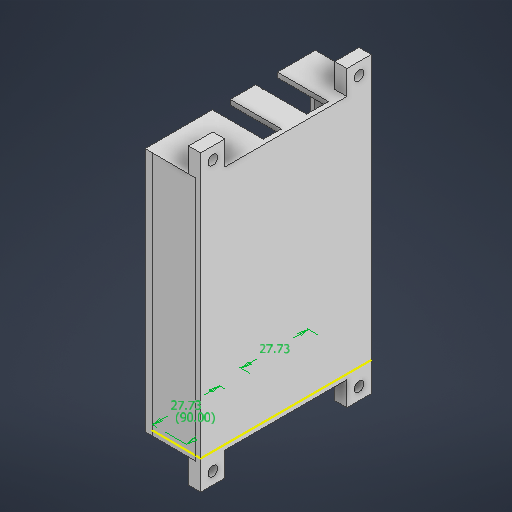
# Autodesk Inventor part: SAFRS-P-0019
Saved by Autodesk Inventor 2026.2 (Build 302298000, 298)
## iProperties
Created: 2025-11-19
Part Number: SAFRS-P-0019
Material: Generic
Document SubType Name: Modeling
Designer: ost97
Density: 1 g/cm^3
Appearance: Default
Author: ost97
Title: STM32 Board
Autodesk Inventor part; units mm, degrees
ref_plane "YZ Plane" through (0, 0, 0) normal (1, 0, 0) x (0, 1, 0)
ref_plane "XZ Plane" through (0, 0, 0) normal (0, 1, 0) x (-1, 0, 0)
ref_plane "XY Plane" through (0, 0, 0) normal (0, 0, 1) x (1, 0, 0)
sketch "Sketch1" plane through (0, 0, 0) normal (0, 1, 0) x (-1, 0, 0)
  line L0 (15, 35.0917) -> (15, 35.175)
  line L1 (-2, 35.175) -> (-2, -33.075)
  line L2 (-2, -33.075) -> (-2, -35.075)
  line L3 (15, 33.075) -> (15, 28.875)
  line L4 (15, 28.875) -> (0, 28.875)
  line L5 (15, 33.075) -> (18, 33.075)
  line L6 (18, 33.075) -> (18, 35.075)
  line L7 (18, 35.075) -> (0, 35.175)
  line L8 (15, -33.075) -> (15, -28.875)
  line L9 (15, -28.875) -> (0, -28.875)
  line L10 (15, -33.075) -> (18, -33.075)
  line L11 (18, -33.075) -> (18, -35.075)
  line L12 (18, -35.075) -> (0, -35.075)
  line L13 (0, 35.175) -> (-2, 35.175)
  line L14 (0, -35.075) -> (-2, -35.075)
  line L15 (0, 28.875) -> (0, -28.875)
  point P0 (0, 0)
  point P1 (15, 39.275)
  point P2 (-2, -37.275)
  point P3 (-2, -39.275)
  point P4 (18, -39.275)
  point P5 (18, -37.275)
  constraints: 32 end point, 7 perpendicular, 5 point on line, 2 horizontal, 2 vertical, 1 midpoint
extrude "Extrusion1" add sketch "Sketch1" against normal blind 97
sketch "Sketch2" plane through (0, 0, 0) normal (0, 1, 0) x (1, 0, 0)
  line L0 (2, 39.275) -> (-18, 39.275) projected
  line L1 (2, -35.175) -> (2, 35.075) projected
  line L2 (-18, 39.275) -> (-18, 37.275) projected
  line L3 (-18, 35.075) -> (-18, 25.675)
  line L4 (0, -28.875) -> (0, 28.875) projected
  line L5 (0, 25.675) -> (0, 17.695)
  line L6 (-18.0003, 10.5) -> (-18.0012, 7.2)
  line L7 (-18, -35.075) -> (-18.0067, -12.57)
  line L8 (-18, -33.075) -> (-18, -35.075) projected
  line L9 (-18, -35.075) -> (0, -35.175) projected
  line L10 (2, 35.075) -> (-18, 35.075) projected
  line L11 (-18, 35.075) -> (-18, 33.075) projected
  line L12 (-18, -35.075) -> (-18, -33.075) projected
  line L13 (-18, -35.075) -> (-18, -10.375)
  line L14 (-18, 33.075) -> (-18, 19.475)
  line L15 (-18, 19.475) -> (0, 19.475)
  line L16 (0, 19.475) -> (0, 11.495)
  line L17 (-18, 10.5) -> (-18, 1)
  line L18 (-18, -33.075) -> (-18.0079, -8.375)
  line L19 (-18.0079, -8.375) -> (0, -8.375)
  line L20 (0, 11.495) -> (0, 10.495)
  line L21 (0, 10.495) -> (-18, 10.5)
  line L22 (-18, 1) -> (-18, 0)
  line L23 (-18, 0) -> (0, 0)
  line L24 (0, -35.175) -> (-18, -35.075) projected
  line L25 (-18, -33.075) -> (-15, -33.075) projected
  line L26 (-18, -35.075) -> (0, -35.175) projected
  line L27 (0, -35.175) -> (2, -35.175) projected
  line L28 (2, -35.175) -> (2, 35.075) projected
  line L29 (2, 35.075) -> (-18, 35.075) projected
  line L30 (-18, 35.075) -> (-18, 33.075) projected
  line L31 (-18, 33.075) -> (-15, 33.075) projected
  line L32 (-15, 33.075) -> (-15, 28.875) projected
  line L33 (-15, 28.875) -> (0, 28.875) projected
  line L34 (0, 28.875) -> (0, -28.875) projected
  line L35 (0, -28.875) -> (-15, -28.875) projected
  line L36 (-15, -28.875) -> (-15, -33.075) projected
  line L37 (-15, -33.075) -> (-18, -33.075) projected
  line L38 (-18, -33.075) -> (-18, -35.075) projected
  line L39 (2, -35.175) -> (2, 35.075) projected
  line L40 (2, 35.075) -> (2, -35.175) projected
  line L41 (-15, -33.075) -> (-18, -33.075) projected
  line L42 (-15, -28.875) -> (-15, -33.075) projected
  line L43 (0, -28.875) -> (-15, -28.875) projected
  line L44 (0, 28.875) -> (0, -28.875) projected
  line L45 (0, 28.875) -> (0, -28.875) projected
  line L46 (0, -28.875) -> (0, 28.875) projected
  line L47 (2, 35.075) -> (-18, 35.075) projected
  line L48 (-18, 35.075) -> (2, 35.075) projected
  line L49 (-15, 28.875) -> (0, 28.875) projected
  line L50 (-15, 28.875) -> (0, 28.875) projected
  line L51 (0, 28.875) -> (-15, 28.875) projected
  line L52 (-15, 33.075) -> (-15, 28.875) projected
  line L53 (-15, 33.075) -> (-15, 28.875) projected
  line L54 (-15, 28.875) -> (-15, 33.075) projected
  line L55 (-18, 35.075) -> (-18, 33.075) projected
  line L56 (-18, 33.075) -> (-18, 35.075) projected
  line L57 (-18, 33.075) -> (-15, 33.075) projected
  line L58 (-15, 33.075) -> (-18, 33.075) projected
  line L59 (-18, 33.075) -> (-15, 33.075) projected
  line L60 (-15, 33.075) -> (-18, 33.075) projected
  line L61 (-18, 33.075) -> (-18, 35.075) projected
  line L62 (0, 28.875) -> (-15, 28.875) projected
  line L63 (-15, -28.875) -> (0, -28.875) projected
  line L64 (-15, -33.075) -> (-15, -28.875) projected
  line L65 (2, 35.075) -> (2, -35.175) projected
  line L66 (0, -35.175) -> (-18, -35.075) projected
  line L67 (-18, -35.075) -> (-18, -33.075) projected
  line L68 (-18, -33.075) -> (-15, -33.075) projected
  line L69 (-15, -33.075) -> (-15, -28.875) projected
  line L70 (-15, -28.875) -> (0, -28.875) projected
  line L71 (0, -28.875) -> (0, 28.875) projected
  line L72 (0, 28.875) -> (-15, 28.875) projected
  line L73 (-15, 28.875) -> (-15, 33.075) projected
  line L74 (-15, 33.075) -> (-18, 33.075) projected
  line L75 (-18, 33.075) -> (-18, 35.075) projected
  line L76 (-18, 35.075) -> (2, 35.075) projected
  line L77 (2, 35.075) -> (2, -35.175) projected
  line L78 (2, -35.175) -> (0, -35.175) projected
  line L79 (-18, 35.075) -> (2, 35.075) projected
  line L80 (-15, 28.875) -> (-15, 33.075) projected
  line L81 (0, -28.875) -> (-15, -28.875) projected
  line L82 (-15, -28.875) -> (0, -28.875) projected
  line L83 (-15, -28.875) -> (-15, -33.075) projected
  line L84 (-15, -33.075) -> (-15, -28.875) projected
  line L85 (2, -35.175) -> (0, -35.175) projected
  line L86 (0, -35.175) -> (2, -35.175) projected
  line L87 (0, -35.175) -> (2, -35.175) projected
  line L88 (2, -35.175) -> (0, -35.175) projected
  line L89 (-18, -35.075) -> (0, -35.175) projected
  line L90 (0, -35.175) -> (-18, -35.075) projected
  line L91 (-15, -33.075) -> (-18, -33.075) projected
  line L92 (-18, -33.075) -> (-15, -33.075) projected
  line L93 (-18, -33.075) -> (-18, -35.075) projected
  line L94 (-18, -35.075) -> (-18, -33.075) projected
  point P0 (0, 33.075)
  point P1 (-18.0067, -12.57)
  dimension "d20" = 13.6
  dimension "d23" = 24.7
  constraints: 28 end point, 6 point on line, 3 vertical, 2 horizontal, 2 perpendicular, 1 collinear, 18 other
  measures "d20" distance of L11.end L14.end
  measures "d23" distance of L8.start L18.end
sketch "Sketch3" plane through (0, -97, 0) normal (0, -1, 0) x (1, 0, 0)
  line L0 (-18, -35.075) -> (2, -35.075) projected
  line L1 (-18, -33.075) -> (-18, -35.075) projected
  line L2 (0, 35.175) -> (-18, 35.075) projected
  line L3 (-18, 35.075) -> (-18, 33.075) projected
  line L4 (-18, -33.075) -> (-18, -5.345)
  line L5 (-18, -5.345) -> (0, -5.345)
  line L6 (-15, 33.075) -> (-18, 33.075) projected
  line L7 (0, 28.875) -> (0, -28.875) projected
  line L8 (-15, 33.075) -> (-15, 28.875) projected
  line L9 (-15, -28.875) -> (-15, -33.075) projected
  line L10 (0, -28.875) -> (-15, -28.875) projected
  line L11 (-15, 28.875) -> (0, 28.875) projected
  line L12 (-18, 33.075) -> (-15, 33.075) projected
  line L13 (-15, -33.075) -> (-18, -33.075) projected
  line L14 (0, 35.175) -> (-18, 35.075) projected
  line L15 (-18, 35.075) -> (-18, 33.075) projected
  line L16 (-18, 33.075) -> (-15, 33.075) projected
  line L17 (-15, 33.075) -> (-15, 28.875) projected
  line L18 (-15, 28.875) -> (0, 28.875) projected
  line L19 (0, 28.875) -> (0, -28.875) projected
  line L20 (0, -28.875) -> (-15, -28.875) projected
  line L21 (-15, -28.875) -> (-15, -33.075) projected
  line L22 (-15, -33.075) -> (-18, -33.075) projected
  line L23 (-18, -33.075) -> (-18, -35.075) projected
  line L24 (-18, -35.075) -> (2, -35.075) projected
  line L25 (2, -35.075) -> (2, 35.175) projected
  line L26 (2, 35.175) -> (0, 35.175) projected
  line L27 (2, 35.175) -> (2, -35.075) projected
  line L28 (2, -35.075) -> (2, 35.175) projected
  line L29 (-18, 35.075) -> (0, 35.175) projected
  line L30 (-18, 33.075) -> (-18, 35.075) projected
  line L31 (2, -35.075) -> (-18, -35.075) projected
  line L32 (-18, -35.075) -> (2, -35.075) projected
  line L33 (-18, -35.075) -> (-18, -33.075) projected
  line L34 (-18, -33.075) -> (-18, -35.075) projected
  line L35 (-15, -33.075) -> (-15, -28.875) projected
  line L36 (-15, -28.875) -> (-15, -33.075) projected
  line L37 (-18, -33.075) -> (-15, -33.075) projected
  line L38 (-15, -33.075) -> (-18, -33.075) projected
  line L39 (-15, -28.875) -> (0, -28.875) projected
  line L40 (0, -28.875) -> (-15, -28.875) projected
  line L41 (0, -28.875) -> (0, 28.875) projected
  line L42 (0, 28.875) -> (0, -28.875) projected
  line L43 (2, -35.075) -> (2, 35.175) projected
  line L44 (2, 35.175) -> (2, -35.075) projected
  line L45 (-18, 35.075) -> (0, 35.175) projected
  line L46 (0, 35.175) -> (2, 35.175) projected
  line L47 (2, 35.175) -> (2, -35.075) projected
  line L48 (2, -35.075) -> (-18, -35.075) projected
  line L49 (-18, -35.075) -> (-18, -33.075) projected
  line L50 (-18, -33.075) -> (-15, -33.075) projected
  line L51 (-15, -33.075) -> (-15, -28.875) projected
  line L52 (-15, -28.875) -> (0, -28.875) projected
  line L53 (0, -28.875) -> (0, 28.875) projected
  line L54 (0, 28.875) -> (-15, 28.875) projected
  line L55 (-15, 28.875) -> (-15, 33.075) projected
  line L56 (-15, 33.075) -> (-18, 33.075) projected
  line L57 (-18, 33.075) -> (-18, 35.075) projected
  line L58 (-15, 28.875) -> (-15, 33.075) projected
  line L59 (0, 28.875) -> (-15, 28.875) projected
  line L60 (0, -28.875) -> (0, 28.875) projected
  line L61 (2, -35.075) -> (-18, -35.075) projected
  line L62 (-15, -28.875) -> (0, -28.875) projected
  line L63 (-15, -33.075) -> (-15, -28.875) projected
  line L64 (-18, -33.075) -> (-15, -33.075) projected
  line L65 (-18, -35.075) -> (-18, -33.075) projected
  line L66 (0, 28.875) -> (-15, 28.875) projected
  line L67 (-15, 28.875) -> (0, 28.875) projected
  line L68 (-15, 28.875) -> (-15, 33.075) projected
  line L69 (-15, 33.075) -> (-15, 28.875) projected
  line L70 (-15, 33.075) -> (-18, 33.075) projected
  line L71 (-18, 33.075) -> (-15, 33.075) projected
  line L72 (-18, 33.075) -> (-18, 35.075) projected
  line L73 (-18, 35.075) -> (-18, 33.075) projected
  line L74 (2, 35.175) -> (0, 35.175) projected
  line L75 (0, 35.175) -> (2, 35.175) projected
  line L76 (0, 35.175) -> (2, 35.175) projected
  line L77 (2, 35.175) -> (0, 35.175) projected
  line L78 (-18, 35.075) -> (0, 35.175) projected
  line L79 (0, 35.175) -> (-18, 35.075) projected
  line L80 (-18, 33.075) -> (-18, 5.345)
  line L81 (-18, 5.345) -> (0, 5.345)
  point P0 (0, 0)
  dimension "d26" = 27.73
  dimension "d33" = 27.73
  dimension "d34" = 90
  constraints: 8 end point, 2 perpendicular, 2 vertical, 1 point on line, 8 other
  measures "d26" distance of L1.start L4.end
  measures "d33" distance of L73.end L80.end
  measures "d34" angle of L6 L80
extrude "Extrusion2" add sketch "Sketch2" along normal blind 2
extrude "Extrusion3" add sketch "Sketch3" along normal blind 2 contours L1 L13 L9 L10 L7 L11 L8 L6 L3 L2 L26 L25 L0 | L4 L5 L7 L10 L9 L13
extrude "Extrusion4" add sketch "Sketch3" along normal up to surface (2 mm away) contours L81 L80 L6 L8 L11 L7
sketch "Sketch5" plane through (-18, 0, -33.075) normal (-1, 0, 0) x (0, 0, 1)
  line L0 (66.15, 2) -> (68.15, 2) projected
  line L1 (68.15, 2) -> (68.25, 2) projected
  line L2 (68.15, 2) -> (68.15, -99) projected
  line L3 (68.25, -99) -> (68.25, 2) projected
  line L4 (68.25, -99) -> (68.25, 2) projected
  line L5 (66.15, 0) -> (66.15, 2) projected
  line L6 (68.25, 2) -> (-2, 2) projected
  line L7 (68.25, -99) -> (68.25, 2) projected
  line L8 (-2, -99) -> (68.25, -99) projected
  line L9 (-2, -99) -> (-2, 2) projected
  line L10 (68.25, 2) -> (-2, 2) projected
  line L11 (38.42, -99) -> (38.42, -97) projected
  line L12 (38.42, -97) -> (61.95, -97) projected
  line L13 (61.95, 0) -> (61.95, -97) projected
  line L14 (41.45, 0) -> (61.95, 0) projected
  line L15 (41.45, 0) -> (41.45, 2) projected
  line L16 (33.075, 2) -> (41.45, 2) projected
  line L17 (33.075, 0) -> (33.075, 2) projected
  line L18 (22.58, 0) -> (33.075, 0) projected
  line L19 (22.58, 0) -> (22.58, 2) projected
  line L20 (13.6, 2) -> (22.58, 2) projected
  line L21 (13.6, 0) -> (13.6, 2) projected
  line L22 (4.2, 0) -> (13.6, 0) projected
  line L23 (4.2, 0) -> (4.2, -97) projected
  line L24 (27.73, -97) -> (4.2, -97) projected
  line L25 (27.73, -97) -> (27.73, -99) projected
  line L26 (38.42, -99) -> (27.73, -99) projected
  line L27 (27.73, -97) -> (27.73, -99) projected
  line L28 (27.73, -97) -> (27.73, -99) projected
  line L29 (27.73, -97) -> (27.73, -99) projected
  line L30 (13.6, 0) -> (13.6, 2) projected
  line L31 (4.2, 0) -> (4.2, -97) projected
  line L32 (4.2, 0) -> (4.2, -97) projected
  line L33 (4.2, 0) -> (4.2, -97) projected
  line L34 (4.2, 0) -> (4.2, -97) projected
  line L35 (27.73, -99) -> (-2, -99) projected
  line L36 (-2, -99) -> (-2, 2) projected
  line L37 (27.73, -99) -> (-2, -99) projected
  line L38 (27.73, -97) -> (27.73, -99) projected
  line L39 (27.73, -97) -> (0, -97) projected
  line L40 (0, 0) -> (0, -97) projected
  line L41 (0, 0) -> (13.6, 0) projected
  line L42 (13.6, 0) -> (13.6, 2) projected
  line L43 (-2, 2) -> (13.6, 2) projected
  line L44 (-2, -99) -> (-2, 2) projected
  line L45 (-2, -99) -> (-2, 2) projected
  line L46 (-2, -99) -> (-2, 2) projected
  line L47 (-2, -99) -> (-2, 2) projected
  line L48 (-2, 2) -> (13.6, 2) projected
  line L49 (0, 0) -> (13.6, 0) projected
  line L50 (0, 0) -> (4.2, 0) projected
  line L51 (0, 0) -> (4.2, 0) projected
  line L52 (0, 0) -> (0, -97) projected
  line L53 (4.2, -97) -> (0, -97) projected
  line L54 (4.2, 0) -> (4.2, -97) projected
  line L55 (0, 0) -> (0, -97) projected
  line L56 (0, 0) -> (0, -97) projected
  line L57 (0, 0) -> (0, -97) projected
  line L58 (0, 0) -> (0, -97) projected
  line L59 (-2, -99) -> (68.25, -99) projected
  line L60 (38.42, -97) -> (61.95, -97) projected
  line L61 (27.73, -97) -> (27.73, -99) projected
  line L62 (38.42, -97) -> (38.42, -99) projected
  line L63 (38.42, -99) -> (38.42, -97) projected
  line L64 (38.42, -97) -> (38.42, -99) projected
  line L65 (38.42, -99) -> (38.42, -97) projected
  line L66 (4.2, -97) -> (0, -97) projected
  line L67 (27.73, -97) -> (0, -97) projected
  line L68 (27.73, -97) -> (4.2, -97) projected
  line L69 (27.73, -97) -> (0, -97) projected
  line L70 (27.73, -97) -> (4.2, -97) projected
  line L71 (4.2, -97) -> (0, -97) projected
  line L72 (61.95, 0) -> (61.95, -97) projected
  line L73 (61.95, 0) -> (61.95, -97) projected
  line L74 (61.95, 0) -> (61.95, -97) projected
  line L75 (61.95, 0) -> (61.95, -97) projected
  line L76 (61.95, -97) -> (66.15, -97) projected
  line L77 (66.15, -97) -> (38.42, -97) projected
  line L78 (61.95, 0) -> (66.15, 0) projected
  line L79 (61.95, -97) -> (66.15, -97) projected
  line L80 (66.15, 0) -> (66.15, -97) projected
  line L81 (61.95, 0) -> (66.15, 0) projected
  line L82 (61.95, 0) -> (61.95, -97) projected
  line L83 (66.15, 0) -> (66.15, -97) projected
  line L84 (66.15, 0) -> (66.15, -97) projected
  line L85 (66.15, 0) -> (66.15, -97) projected
  line L86 (66.15, -97) -> (38.42, -97) projected
  line L87 (61.95, -97) -> (66.15, -97) projected
  line L88 (38.42, -97) -> (61.95, -97) projected
  line L89 (68.15, -99) -> (38.42, -99) projected
  line L90 (66.15, 0) -> (66.15, -97) projected
  line L91 (66.15, -97) -> (38.42, -97) projected
  line L92 (38.42, -97) -> (38.42, -99) projected
  line L93 (68.15, -99) -> (38.42, -99) projected
  line L94 (68.15, 2) -> (68.15, -99) projected
  line L95 (66.15, 2) -> (68.15, 2) projected
  line L96 (66.15, 0) -> (66.15, 2) projected
  line L97 (68.25, -99) -> (68.15, -99) projected
  line L98 (68.15, 2) -> (68.15, -99) projected
  line L99 (68.25, -99) -> (68.15, -99) projected
  line L100 (68.25, -99) -> (68.25, 2) projected
  line L101 (68.15, 2) -> (68.25, 2) projected
  line L102 (68.25, -99) -> (68.25, 2) projected
  line L103 (68.25, -99) -> (68.25, 2) projected
  line L104 (66.15, 0) -> (66.15, -97) projected
  line L105 (13.6, 2) -> (22.58, 2) projected
  line L106 (4.2, 0) -> (13.6, 0) projected
  line L107 (13.6, 0) -> (13.6, 2) projected
  line L108 (41.45, 0) -> (61.95, 0) projected
  line L109 (33.075, 2) -> (41.45, 2) projected
  line L110 (22.58, 0) -> (33.075, 0) projected
  line L111 (22.58, 0) -> (22.58, 2) projected
  line L112 (41.45, 0) -> (41.45, 2) projected
  line L113 (33.075, 0) -> (33.075, 2) projected
  line L114 (38.42, -99) -> (27.73, -99) projected
  line L115 (27.73, -99) -> (-2, -99) projected
  line L116 (-2, -99) -> (68.25, -99) projected
  line L117 (68.25, -99) -> (68.15, -99) projected
  line L118 (68.15, -99) -> (38.42, -99) projected
  line L119 (38.42, -99) -> (27.73, -99) projected
  line L120 (22.58, 2) -> (22.575, 2) projected
  line L121 (22.575, 0) -> (22.575, 2) projected
  line L122 (22.575, 2) -> (33.075, 2) projected
  line L123 (33.075, 0) -> (33.075, 2) projected
  line L124 (41.45, 0) -> (41.45, 2) projected
  line L125 (41.45, 2) -> (66.15, 2) projected
  line L126 (41.45, 0) -> (66.15, 0) projected
  line L127 (22.58, 0) -> (22.575, 0) projected
  line L128 (22.575, 0) -> (33.075, 0) projected
  line L129 (41.45, 0) -> (66.15, 0) projected
  line L130 (41.45, 0) -> (61.95, 0) projected
  line L131 (61.95, 0) -> (66.15, 0) projected
  line L132 (41.45, 0) -> (41.45, 2) projected
  line L133 (41.45, 0) -> (41.45, 2) projected
  line L134 (41.45, 0) -> (66.15, 0) projected
  line L135 (66.15, 0) -> (66.15, 2) projected
  line L136 (41.45, 2) -> (66.15, 2) projected
  line L137 (41.45, 0) -> (41.45, 2) projected
  line L138 (22.58, 2) -> (22.575, 2) projected
  line L139 (22.575, 2) -> (33.075, 2) projected
  line L140 (33.075, 2) -> (41.45, 2) projected
  line L141 (41.45, 2) -> (66.15, 2) projected
  line L142 (66.15, 2) -> (68.15, 2) projected
  line L143 (68.15, 2) -> (68.25, 2) projected
  line L144 (68.25, 2) -> (-2, 2) projected
  line L145 (-2, 2) -> (13.6, 2) projected
  line L146 (13.6, 2) -> (22.58, 2) projected
  line L147 (22.58, 0) -> (33.075, 0) projected
  line L148 (22.575, 0) -> (33.075, 0) projected
  line L149 (22.58, 0) -> (22.575, 0) projected
  line L150 (22.58, 0) -> (22.575, 0) projected
  line L151 (22.575, 0) -> (22.575, 2) projected
  line L152 (22.58, 2) -> (22.575, 2) projected
  line L153 (22.58, 0) -> (22.58, 2) projected
  line L154 (22.575, 0) -> (33.075, 0) projected
  line L155 (33.075, 0) -> (33.075, 2) projected
  line L156 (22.575, 2) -> (33.075, 2) projected
  line L157 (22.575, 0) -> (22.575, 2) projected
  line L158 (13.6, 0) -> (13.6, 2) projected
  line L159 (13.6, 0) -> (13.6, 2) projected
  line L160 (0, 0) -> (4.2, 0) projected
  line L161 (4.2, 0) -> (13.6, 0) projected
  line L162 (0, 0) -> (13.6, 0) projected
  line L163 (33.075, 0) -> (33.075, 2) projected
  line L164 (33.075, 0) -> (33.075, 2) projected
  line L165 (66.15, -97) -> (61.95, -97) projected
  line L166 (61.95, -97) -> (4.2, -97) projected
  line L167 (4.2, -97) -> (61.95, -97) projected
  line L168 (4.2, -97) -> (61.95, -97) projected
  line L169 (61.95, -97) -> (4.2, -97) projected
  line L170 (4.2, -97) -> (61.95, -97) projected
  line L171 (61.95, -97) -> (4.2, -97) projected
  line L172 (66.15, -97) -> (38.42, -97) projected
  line L173 (68.25, -97) -> (68.15, -97) projected
  line L174 (68.15, -97) -> (68.25, -97) projected
  line L175 (68.15, -97) -> (68.25, -97) projected
  line L176 (68.25, -97) -> (68.15, -97) projected
  line L177 (68.15, -97) -> (66.15, -97) projected
  line L178 (68.15, -97) -> (66.15, -97) projected
  line L179 (66.15, -97) -> (68.15, -97) projected
  line L180 (4.2, -97) -> (0, -97) projected
  line L181 (0, -97) -> (27.73, -97) projected
  line L182 (-2, -97) -> (68.25, -97) projected
  line L183 (68.25, -97) -> (-2, -97) projected
  line L184 (-2, -97) -> (68.25, -97) projected
  line L185 (68.25, -97) -> (-2, -97) projected
  line L186 (-2, -97) -> (68.25, -97) projected
  line L187 (68.25, -97) -> (-2, -97) projected
  line L188 (0, -97) -> (-2, -97) projected
  line L189 (0, -97) -> (-2, -97) projected
  line L190 (-2, -97) -> (0, -97) projected
  line L191 (0, -97) -> (-2, -97) projected
  line L192 (4.2, -97) -> (0, -97) projected
  line L193 (0, -97) -> (4.2, -97) projected
  line L194 (4.2, -97) -> (0, -97) projected
  line L195 (66.15, -97) -> (61.95, -97) projected
  line L196 (61.95, -97) -> (66.15, -97) projected
  line L197 (61.95, -97) -> (66.15, -97) projected
  line L198 (-2, -97) -> (0, -97) projected
  line L199 (0, -97) -> (4.2, -97) projected
  line L200 (0, -97) -> (4.2, -97) projected
  line L201 (-2, -97) -> (0, -97) projected
  line L202 (66.15, -97) -> (68.15, -97) projected
  line L203 (68.15, -97) -> (68.25, -97) projected
  line L204 (68.25, -97) -> (68.15, -97) projected
  line L205 (61.95, -97) -> (66.15, -97) projected
  line L206 (66.15, -97) -> (61.95, -97) projected
  line L207 (66.15, -97) -> (68.15, -97) projected
  line L208 (68.15, -97) -> (66.15, -97) projected
  point P0 (33.075, -97)
  point P1 (-2, 2)
  constraints: 2 coincident, 1 horizontal alignment, 1 perpendicular, 61 other
extrude "Extrusion5" add sketch "Sketch5" along normal blind 3 contours L0 L2 L177 L80 L5 | L5 L78 L14 L15 L6 | L2 L8 L11 L12 L76 L177 | L17 L18 L19 L6 | L8 L9 L182 L39 L24 L25 | L21 L22 L41 L40 L182 L9 L6
sketch "Sketch6" plane through (0, 2, 0) normal (0, 1, 0) x (1, 0, 0)
  line L0 (0, 0) -> (0, -8.375) projected
  line L1 (0, -8.375) -> (-21, -8.375) projected
  line L2 (0, -8.375) -> (0, -7.375)
  line L3 (0, -7.375) -> (-21, -7.375)
  line L4 (-21, -7.375) -> (-21, -8.375)
  dimension "d39" = 1
  constraints: 6 end point, 2 perpendicular, 1 point on line
  measures "d39" distance of L0.end L2.end
extrude "Extrusion6" add sketch "Sketch6" against normal up to surface (2 mm away)
sketch "스케치7" plane through (2, 2, 35.175) normal (1, 0, 0) x (0, 0, -1)
  line L0 (0, -101) -> (0, 0) projected
  line L1 (70.25, -101) -> (0, -101) projected
  line L2 (70.25, -101) -> (70.25, 0) projected
  line L3 (0, 0) -> (70.25, 0) projected
  line L4 (70.25, -101) -> (60.25, -101)
  line L5 (60.25, -101) -> (60.25, -111)
  line L6 (60.25, -111) -> (70.25, -111)
  line L7 (70.25, -111) -> (70.25, -101)
  line L8 (70.25, -50.5) -> (0, -50.5) construction
  line L9 (35.125, 0) -> (35.125, -101) construction
  line L10 (60.25, 0) -> (60.25, 10)
  line L11 (60.25, 10) -> (70.25, 10)
  line L12 (70.25, 10) -> (70.25, 0)
  line L13 (10, -101) -> (10, -111)
  line L14 (10, -111) -> (0, -111)
  line L15 (0, -111) -> (0, -101)
  line L16 (10, 0) -> (10, 10)
  line L17 (10, 10) -> (0, 10)
  line L18 (0, 10) -> (0, 0)
  circle A0 centre (65.25, -106) radius 2
  circle A1 centre (65.25, 5) radius 2
  circle A2 centre (5, -106) radius 2
  circle A3 centre (5, 5) radius 2
  point P0 (35.175, -2)
  point P1 (10, 0)
  dimension "d42" = 10
  dimension "d43" = 10
  dimension "d44" = 4
  dimension "d45" = 111
  dimension "d46" = 60.25
  constraints: 30 end point, 12 symmetric about line, 4 centre point, 4 midpoint, 2 parallel, 1 horizontal, 1 perpendicular, 3 other
  measures "d42" distance of L6.end L1.start
  measures "d43" distance of L5.end L6.end
  measures "d44" diameter of A0
  measures "d45" distance of A1.centre A0.centre
  measures "d46" distance of A2.centre A0.centre
extrude "돌출7" add sketch "스케치7" against normal blind 5 contours L1 L13 L14 L15 | L18 L17 L16 L3 | L1 L7 L6 L5 | L10 L11 L12 L3
body "Solid1"
